Autodesk Inventor part; units mm, degrees
(part 2 of 2)
sketch "Sketch3" plane through (0, 0, 0.5) normal (0, 0, 1) x (1, 0, 0)
  line L0 (157.5, 62.5) -> (-51.75, 62.5) projected
  line L1 (-51.75, 62.5) -> (-51.75, 14.7) projected
  line L2 (-51.75, 14.7) -> (-42, 14.7) projected
  line L3 (-42, 14.7) -> (-42, -4.9) projected
  line L4 (-42, -4.9) -> (-56.25, -4.9) projected
  line L5 (-56.25, -4.9) -> (-56.25, -23.5) projected
  line L6 (-56.25, -23.5) -> (67, -23.5) projected
  line L7 (67, -23.5) -> (67, -42.6375) projected
  line L8 (67, -42.6375) -> (80, -42.6375) projected
  line L9 (80, -42.6375) -> (80, -62.5) projected
  line L10 (80, -62.5) -> (157.5, -62.5) projected
  line L11 (157.5, -62.5) -> (157.5, -41.5) projected
  line L12 (157.5, -41.5) -> (139.5, -41.5) projected
  line L13 (139.5, -41.5) -> (139.5, 12.5) projected
  line L14 (139.5, 12.5) -> (157.5, 12.5) projected
  line L15 (157.5, 12.5) -> (157.5, 62.5) projected
  line L16 (119.95, -13.75) -> (132.35, -13.75) projected
  line L17 (132.35, -13.75) -> (132.35, -19.8) projected
  line L18 (132.35, -19.8) -> (119.95, -19.8) projected
  line L19 (119.95, -19.8) -> (119.95, -13.75) projected
  line L20 (119.95, 10.25) -> (132.35, 10.25) projected
  line L21 (132.35, 10.25) -> (132.35, 4.2) projected
  line L22 (132.35, 4.2) -> (119.95, 4.2) projected
  line L23 (119.95, 4.2) -> (119.95, 10.25) projected
  line L24 (-35.025, -21.225) -> (-35.025, -7.175) projected
  line L25 (-35.025, -7.175) -> (-20.975, -7.175) projected
  line L26 (-20.975, -7.175) -> (-20.975, -21.225) projected
  line L27 (-20.975, -21.225) -> (-35.025, -21.225) projected
  line L28 (-54.025, -7.175) -> (-39.975, -7.175) projected
  line L29 (-39.975, -7.175) -> (-39.975, -21.225) projected
  line L30 (-39.975, -21.225) -> (-54.025, -21.225) projected
  line L31 (-54.025, -21.225) -> (-54.025, -7.175) projected
  line L32 (-25.725, 11.925) -> (-25.725, -2.125) projected
  line L33 (-25.725, -2.125) -> (-39.775, -2.125) projected
  line L34 (-39.775, -2.125) -> (-39.775, 11.925) projected
  line L35 (-39.775, 11.925) -> (-25.725, 11.925) projected
  line L36 (-20.775, 11.925) -> (-6.725, 11.925) projected
  line L37 (-6.725, 11.925) -> (-6.725, -2.125) projected
  line L38 (-6.725, -2.125) -> (-20.775, -2.125) projected
  line L39 (-20.775, -2.125) -> (-20.775, 11.925) projected
  line L40 (-1.775, 11.925) -> (12.275, 11.925) projected
  line L41 (12.275, 11.925) -> (12.275, -2.125) projected
  line L42 (12.275, -2.125) -> (-1.775, -2.125) projected
  line L43 (-1.775, -2.125) -> (-1.775, 11.925) projected
  line L44 (-1.975, -7.175) -> (-1.975, -21.225) projected
  line L45 (-1.975, -21.225) -> (-16.025, -21.225) projected
  line L46 (-16.025, -21.225) -> (-16.025, -7.175) projected
  line L47 (-16.025, -7.175) -> (-1.975, -7.175) projected
  line L48 (2.975, -7.175) -> (17.025, -7.175) projected
  line L49 (17.025, -7.175) -> (17.025, -21.225) projected
  line L50 (17.025, -21.225) -> (2.975, -21.225) projected
  line L51 (2.975, -21.225) -> (2.975, -7.175) projected
  line L52 (119.45, 2.25) -> (133.5, 2.25) projected
  line L53 (133.5, 2.25) -> (133.5, -11.8) projected
  line L54 (133.5, -11.8) -> (119.45, -11.8) projected
  line L55 (119.45, -11.8) -> (119.45, 2.25) projected
  line L56 (83.725, -45.45) -> (97.775, -45.45) projected
  line L57 (97.775, -45.45) -> (97.775, -59.5) projected
  line L58 (97.775, -59.5) -> (83.725, -59.5) projected
  line L59 (83.725, -59.5) -> (83.725, -45.45) projected
  line L60 (102.725, -45.45) -> (116.775, -45.45) projected
  line L61 (116.775, -45.45) -> (116.775, -59.5) projected
  line L62 (116.775, -59.5) -> (102.725, -59.5) projected
  line L63 (102.725, -59.5) -> (102.725, -45.45) projected
  line L64 (135.775, -45.45) -> (135.775, -59.5) projected
  line L65 (135.775, -59.5) -> (121.725, -59.5) projected
  line L66 (121.725, -59.5) -> (121.725, -45.45) projected
  line L67 (121.725, -45.45) -> (135.775, -45.45) projected
  line L68 (140.725, -45.45) -> (154.775, -45.45) projected
  line L69 (154.775, -45.45) -> (154.775, -59.5) projected
  line L70 (154.775, -59.5) -> (140.725, -59.5) projected
  line L71 (140.725, -59.5) -> (140.725, -45.45) projected
  line L72 (121.725, -40.325) -> (121.725, -26.275) projected
  line L73 (121.725, -26.275) -> (135.775, -26.275) projected
  line L74 (135.775, -26.275) -> (135.775, -40.325) projected
  line L75 (135.775, -40.325) -> (121.725, -40.325) projected
  line L76 (95.475, -40.325) -> (95.475, -26.275) projected
  line L77 (95.475, -26.275) -> (109.525, -26.275) projected
  line L78 (109.525, -26.275) -> (109.525, -40.325) projected
  line L79 (109.525, -40.325) -> (95.475, -40.325) projected
  line L80 (69.225, -26.275) -> (83.275, -26.275) projected
  line L81 (83.275, -26.275) -> (83.275, -40.325) projected
  line L82 (83.275, -40.325) -> (69.225, -40.325) projected
  line L83 (69.225, -40.325) -> (69.225, -26.275) projected
  line L84 (97.975, -7.175) -> (112.025, -7.175) projected
  line L85 (112.025, -7.175) -> (112.025, -21.225) projected
  line L86 (112.025, -21.225) -> (97.975, -21.225) projected
  line L87 (97.975, -21.225) -> (97.975, -7.175) projected
  line L88 (78.975, -7.175) -> (93.025, -7.175) projected
  line L89 (93.025, -7.175) -> (93.025, -21.225) projected
  line L90 (93.025, -21.225) -> (78.975, -21.225) projected
  line L91 (78.975, -21.225) -> (78.975, -7.175) projected
  line L92 (59.975, -21.225) -> (59.975, -7.175) projected
  line L93 (59.975, -7.175) -> (74.025, -7.175) projected
  line L94 (74.025, -7.175) -> (74.025, -21.225) projected
  line L95 (74.025, -21.225) -> (59.975, -21.225) projected
  line L96 (40.975, -7.175) -> (55.025, -7.175) projected
  line L97 (55.025, -7.175) -> (55.025, -21.225) projected
  line L98 (55.025, -21.225) -> (40.975, -21.225) projected
  line L99 (40.975, -21.225) -> (40.975, -7.175) projected
  line L100 (21.975, -7.175) -> (36.025, -7.175) projected
  line L101 (36.025, -7.175) -> (36.025, -21.225) projected
  line L102 (36.025, -21.225) -> (21.975, -21.225) projected
  line L103 (21.975, -21.225) -> (21.975, -7.175) projected
  line L104 (93.225, -2.125) -> (93.225, 11.925) projected
  line L105 (93.225, 11.925) -> (107.275, 11.925) projected
  line L106 (107.275, 11.925) -> (107.275, -2.125) projected
  line L107 (107.275, -2.125) -> (93.225, -2.125) projected
  line L108 (74.225, 11.925) -> (88.275, 11.925) projected
  line L109 (88.275, 11.925) -> (88.275, -2.125) projected
  line L110 (88.275, -2.125) -> (74.225, -2.125) projected
  line L111 (74.225, -2.125) -> (74.225, 11.925) projected
  line L112 (55.225, 11.925) -> (69.275, 11.925) projected
  line L113 (69.275, 11.925) -> (69.275, -2.125) projected
  line L114 (69.275, -2.125) -> (55.225, -2.125) projected
  line L115 (55.225, -2.125) -> (55.225, 11.925) projected
  line L116 (36.225, 11.925) -> (50.275, 11.925) projected
  line L117 (50.275, 11.925) -> (50.275, -2.125) projected
  line L118 (50.275, -2.125) -> (36.225, -2.125) projected
  line L119 (36.225, -2.125) -> (36.225, 11.925) projected
  line L120 (17.225, 11.925) -> (31.275, 11.925) projected
  line L121 (31.275, 11.925) -> (31.275, -2.125) projected
  line L122 (31.275, -2.125) -> (17.225, -2.125) projected
  line L123 (17.225, -2.125) -> (17.225, 11.925) projected
  line L124 (140.475, 31.025) -> (154.525, 31.025) projected
  line L125 (154.525, 31.025) -> (154.525, 16.975) projected
  line L126 (154.525, 16.975) -> (140.475, 16.975) projected
  line L127 (140.475, 16.975) -> (140.475, 31.025) projected
  line L128 (121.475, 31.025) -> (135.525, 31.025) projected
  line L129 (135.525, 31.025) -> (135.525, 16.975) projected
  line L130 (135.525, 16.975) -> (121.475, 16.975) projected
  line L131 (121.475, 16.975) -> (121.475, 31.025) projected
  line L132 (102.475, 31.025) -> (116.525, 31.025) projected
  line L133 (116.525, 31.025) -> (116.525, 16.975) projected
  line L134 (116.525, 16.975) -> (102.475, 16.975) projected
  line L135 (102.475, 16.975) -> (102.475, 31.025) projected
  line L136 (83.475, 16.975) -> (83.475, 31.025) projected
  line L137 (83.475, 31.025) -> (97.525, 31.025) projected
  line L138 (97.525, 31.025) -> (97.525, 16.975) projected
  line L139 (97.525, 16.975) -> (83.475, 16.975) projected
  line L140 (64.475, 31.025) -> (78.525, 31.025) projected
  line L141 (78.525, 31.025) -> (78.525, 16.975) projected
  line L142 (78.525, 16.975) -> (64.475, 16.975) projected
  line L143 (64.475, 16.975) -> (64.475, 31.025) projected
  line L144 (45.475, 31.025) -> (59.525, 31.025) projected
  line L145 (59.525, 31.025) -> (59.525, 16.975) projected
  line L146 (59.525, 16.975) -> (45.475, 16.975) projected
  line L147 (45.475, 16.975) -> (45.475, 31.025) projected
  line L148 (26.475, 31.025) -> (40.525, 31.025) projected
  line L149 (40.525, 31.025) -> (40.525, 16.975) projected
  line L150 (40.525, 16.975) -> (26.475, 16.975) projected
  line L151 (26.475, 16.975) -> (26.475, 31.025) projected
  line L152 (138.975, 45.475) -> (138.975, 59.525) projected
  line L153 (138.975, 59.525) -> (153.025, 59.525) projected
  line L154 (153.025, 59.525) -> (153.025, 45.475) projected
  line L155 (153.025, 45.475) -> (138.975, 45.475) projected
  line L156 (105.475, 45.475) -> (105.475, 59.525) projected
  line L157 (105.475, 59.525) -> (119.525, 59.525) projected
  line L158 (119.525, 59.525) -> (119.525, 45.475) projected
  line L159 (119.525, 45.475) -> (105.475, 45.475) projected
  line L160 (81.475, 59.525) -> (95.525, 59.525) projected
  line L161 (95.525, 59.525) -> (95.525, 45.475) projected
  line L162 (95.525, 45.475) -> (81.475, 45.475) projected
  line L163 (81.475, 45.475) -> (81.475, 59.525) projected
  line L164 (57.475, 45.475) -> (57.475, 59.525) projected
  line L165 (57.475, 59.525) -> (71.525, 59.525) projected
  line L166 (71.525, 59.525) -> (71.525, 45.475) projected
  line L167 (71.525, 45.475) -> (57.475, 45.475) projected
  line L168 (33.475, 59.525) -> (47.525, 59.525) projected
  line L169 (47.525, 59.525) -> (47.525, 45.475) projected
  line L170 (47.525, 45.475) -> (33.475, 45.475) projected
  line L171 (33.475, 45.475) -> (33.475, 59.525) projected
  line L172 (21.525, 16.975) -> (7.475, 16.975) projected
  line L173 (7.475, 16.975) -> (7.475, 31.025) projected
  line L174 (7.475, 31.025) -> (21.525, 31.025) projected
  line L175 (21.525, 31.025) -> (21.525, 16.975) projected
  line L176 (-11.525, 16.975) -> (-11.525, 31.025) projected
  line L177 (-11.525, 31.025) -> (2.525, 31.025) projected
  line L178 (2.525, 31.025) -> (2.525, 16.975) projected
  line L179 (2.525, 16.975) -> (-11.525, 16.975) projected
  line L180 (-16.475, 16.975) -> (-30.525, 16.975) projected
  line L181 (-30.525, 16.975) -> (-30.525, 31.025) projected
  line L182 (-30.525, 31.025) -> (-16.475, 31.025) projected
  line L183 (-16.475, 31.025) -> (-16.475, 16.975) projected
  line L184 (-49.525, 31.025) -> (-35.475, 31.025) projected
  line L185 (-35.475, 31.025) -> (-35.475, 16.975) projected
  line L186 (-35.475, 16.975) -> (-49.525, 16.975) projected
  line L187 (-49.525, 16.975) -> (-49.525, 31.025) projected
  line L188 (-32.975, 59.525) -> (-32.975, 45.475) projected
  line L189 (-32.975, 45.475) -> (-47.025, 45.475) projected
  line L190 (-47.025, 45.475) -> (-47.025, 59.525) projected
  line L191 (-47.025, 59.525) -> (-32.975, 59.525) projected
  line L192 (-23.025, 59.525) -> (-8.975, 59.525) projected
  line L193 (-8.975, 59.525) -> (-8.975, 45.475) projected
  line L194 (-8.975, 45.475) -> (-23.025, 45.475) projected
  line L195 (-23.025, 45.475) -> (-23.025, 59.525) projected
  line L196 (23.525, 45.475) -> (9.475, 45.475) projected
  line L197 (9.475, 45.475) -> (9.475, 59.525) projected
  line L198 (9.475, 59.525) -> (23.525, 59.525) projected
  line L199 (23.525, 59.525) -> (23.525, 45.475) projected
  line L200 (-38.5, 42.5) -> (6.5, 42.5) projected
  line L201 (6.5, 42.5) -> (6.5, 33.5) projected
  line L202 (6.5, 33.5) -> (-38.5, 33.5) projected
  line L203 (-38.5, 33.5) -> (-38.5, 42.5) projected
  line L204 (135.475, 61.525) -> (156.525, 61.525)
  line L205 (156.525, 61.525) -> (156.525, 43.475)
  line L206 (156.525, 43.475) -> (135.475, 43.475)
  line L207 (135.475, 43.475) -> (135.475, 61.525)
  line L208 (123.025, 61.525) -> (5.975, 61.525)
  line L209 (5.975, 61.525) -> (5.975, 43.475)
  line L210 (5.975, 43.475) -> (123.025, 43.475)
  line L211 (123.025, 43.475) -> (123.025, 61.525)
  line L212 (-5.475, 61.525) -> (-51.75, 61.525)
  line L213 (-51.75, 61.525) -> (-51.75, 43.475)
  line L214 (-51.75, 43.475) -> (-5.475, 43.475)
  line L215 (-5.475, 43.475) -> (-5.475, 61.525)
  line L216 (-51.75, 33.025) -> (156.525, 33.025)
  line L217 (156.525, 33.025) -> (156.525, 14.975)
  line L218 (156.525, 14.975) -> (138.5, 14.975)
  line L219 (138.5, 14.975) -> (138.5, -43.45)
  line L220 (138.5, -43.45) -> (157.5, -43.45)
  point P0 (0, 0)
  dimension "d27" = 3.5
  dimension "d28" = 2
  dimension "d29" = 2
  dimension "d30" = 3.5
  dimension "d31" = 3.5
  dimension "d32" = 3.5
  dimension "d33" = 3.5
  dimension "d34" = 2
  dimension "d36" = 2
  dimension "d37" = 5
  dimension "d38" = 2
  constraints: 34 end point, 7 parallel, 7 perpendicular, 5 point on line, 3 collinear, 3 horizontal
  measures "d27" distance between parallel lines of L205 L154
  measures "d28" distance between parallel lines of L204 L153
  measures "d29" distance between parallel lines of L206 L155
  measures "d30" distance between parallel lines of L152 L207
  measures "d31" distance between parallel lines of L211 L158
  measures "d32" distance between parallel lines of L197 L209
  measures "d33" distance between parallel lines of L193 L215
  measures "d34" distance between parallel lines of L216 L124
  measures "d36" distance between parallel lines of L218 L126
  measures "d37" distance between parallel lines of L219 L53
  measures "d38" distance between parallel lines of L220 L68
extrude "Extrusion3" add sketch "Sketch3" along normal blind 2.5 contours L212 L215 L214 L1 | L216 L217 L218 L219 L220 L11 L10 L9 L8 L7 L6 L5 L4 L3 L2 L1 | L204 L205 L206 L207 | L211 L210 L209 L208
sketch "Sketch4" plane through (0, 0, 0) normal (0, 0, -1) x (-1, 0, 0)
  line L0 (-135, 10.25) -> (-117.95, 10.25) construction
  line L1 (-117.95, 4.2) -> (-135, 4.2) construction
  line L2 (-135, -13.75) -> (-117.95, -13.75) construction
  line L3 (-117.95, -19.8) -> (-135, -19.8) construction
  line L4 (-116.95, 10.25) -> (-134.35, 10.25)
  line L5 (-134.35, 10.25) -> (-134.35, 4.2)
  line L6 (-134.35, 4.2) -> (-123.95, 4.2)
  line L7 (-116.95, 4.2) -> (-116.95, 10.25)
  line L8 (-123.95, -13.75) -> (-134.35, -13.75)
  line L9 (-134.35, -13.75) -> (-134.35, -19.8)
  line L10 (-134.35, -19.8) -> (-116.95, -19.8)
  line L11 (-116.95, -19.8) -> (-116.95, -13.75)
  line L12 (-123.95, 4.2) -> (-123.95, -13.75)
  line L13 (-116.95, 4.2) -> (-116.95, -13.75)
  line L14 (-132.35, 10.25) -> (-132.35, 4.2) construction
  line L15 (-119.95, 4.2) -> (-119.95, 10.25) projected
  point P0 (0, 0)
  dimension "d41" = 2
  dimension "d42" = 3
  dimension "d43" = 4
  constraints: 20 end point, 4 parallel, 4 point on line, 3 collinear, 3 perpendicular, 2 horizontal
  measures "d41" distance between parallel lines of L5 L14
  measures "d42" distance between parallel lines of L7 L15
  measures "d43" distance between parallel lines of L12 L15
extrude "Extrusion4" cut sketch "Sketch4" against normal blind 2
equation "\"d0\" = dpg"
equation "\"d1\" = dpg"
equation "\"d2\" = dpg"
equation "\"d3\" = dpg"
equation "\"d4\" = 0.5 * dpg"
equation "\"d5\" = 0.5 * dpg"
equation "\"d6\" = 0.5 * dpg"
equation "\"d7\" = 0.5 * dpg"
equation "\"d8\" = 0.5 * dpg"
equation "\"d29\" = d28"
equation "\"d30\" = d27"
equation "\"d31\" = d27"
equation "\"d32\" = d27"
equation "\"d33\" = d27"
equation "\"d34\" = d28"
equation "\"d36\" = d28"
equation "\"d38\" = d28"
equation "\"dpg\" = 0.5"
body "Solid2"
